Autodesk Fusion 360 part; units mm, degrees
(part 4 of 7)
  spline S86 degree 3 poles (7.7647, -28.9777) (7.9861, -28.9172) (8.1489, -28.7875) (8.2245, -28.6924) (8.2561, -28.6527) (8.2762, -28.616) (8.2885, -28.5883) (8.2955, -28.5727) (8.3002, -28.5603) (8.3276, -28.4858) (8.3447, -28.4393) (8.3614, -28.3763) (8.4396, -28.2255) (8.4953, -28.1181) (8.6034, -27.9308) (8.8139, -27.7502) (8.9794, -27.6083) (9.1711, -27.5171) (9.2695, -27.4797) (9.36, -27.4454) (9.4336, -27.4171) (9.6094, -27.3931) (9.8296, -27.363) (10.1211, -27.3993) (10.2894, -27.4529) (10.6015, -27.5525) (10.6588, -27.6214) (10.7168, -27.6578) (10.8456, -27.7385) (10.8244, -27.7262) (10.8574, -27.741) (10.9657, -27.7894) (11.2076, -27.8277) (11.4806, -27.7163) knots 0.001251 0.001251 0.001251 0.001251 0.25 0.25 0.25 0.35404 0.35404 0.35404 0.412746 0.412746 0.412746 0.449449 0.449449 0.449449 0.475576 0.475576 0.475576 0.496118 0.496118 0.496118 0.514995 0.514995 0.514995 0.538647 0.538647 0.538647 0.582499 0.582499 0.582499 0.679826 0.679826 0.679826 0.99875 0.99875 0.99875 0.99875
  spline S87 degree 3 poles (11.4806, -27.7163) (11.6922, -27.6274) (11.8368, -27.4775) (11.8992, -27.3735) (11.9254, -27.3299) (11.9405, -27.2909) (11.9492, -27.2619) (11.954, -27.2455) (11.9571, -27.2325) (11.9745, -27.1552) (11.9853, -27.1068) (11.9937, -27.0422) (12.0516, -26.8824) (12.0928, -26.7687) (12.1755, -26.5688) (12.3606, -26.3624) (12.5062, -26.2) (12.6843, -26.0846) (12.7771, -26.0347) (12.8623, -25.9889) (12.9316, -25.9512) (13.1027, -25.9045) (13.3171, -25.8459) (13.6108, -25.8438) (13.7847, -25.875) (14.1071, -25.933) (14.173, -25.9939) (14.2352, -26.0223) (14.3734, -26.0856) (14.3508, -26.0762) (14.3854, -26.0865) (14.4991, -26.1203) (14.744, -26.1267) (15.0001, -25.9807) knots 0.001251 0.001251 0.001251 0.001251 0.25 0.25 0.25 0.35404 0.35404 0.35404 0.412746 0.412746 0.412746 0.449449 0.449449 0.449449 0.475576 0.475576 0.475576 0.496118 0.496118 0.496118 0.514995 0.514995 0.514995 0.538647 0.538647 0.538647 0.582499 0.582499 0.582499 0.679826 0.679826 0.679826 0.99875 0.99875 0.99875 0.99875
  spline S88 degree 3 poles (15.0001, -25.9807) (15.1983, -25.8649) (15.322, -25.6975) (15.3704, -25.5861) (15.3906, -25.5395) (15.4006, -25.4989) (15.4053, -25.469) (15.408, -25.4521) (15.4093, -25.4388) (15.4165, -25.3599) (15.421, -25.3105) (15.4208, -25.2453) (15.4573, -25.0794) (15.4834, -24.9613) (15.5393, -24.7523) (15.6959, -24.5234) (15.819, -24.3435) (15.9805, -24.2058) (16.066, -24.1443) (16.1444, -24.0877) (16.2082, -24.0413) (16.3718, -23.9726) (16.5767, -23.8866) (16.8677, -23.8461) (17.0441, -23.8544) (17.3713, -23.8698) (17.4446, -23.9215) (17.51, -23.9416) (17.6553, -23.9863) (17.6316, -23.9799) (17.6673, -23.9856) (17.7844, -24.0044) (18.028, -23.9787) (18.2629, -23.8005) knots 0.001251 0.001251 0.001251 0.001251 0.25 0.25 0.25 0.35404 0.35404 0.35404 0.412746 0.412746 0.412746 0.449449 0.449449 0.449449 0.475576 0.475576 0.475576 0.496118 0.496118 0.496118 0.514995 0.514995 0.514995 0.538647 0.538647 0.538647 0.582499 0.582499 0.582499 0.679826 0.679826 0.679826 0.99875 0.99875 0.99875 0.99875
  spline S89 degree 3 poles (18.2629, -23.8005) (18.4443, -23.6598) (18.5451, -23.4777) (18.5786, -23.361) (18.5925, -23.3122) (18.5971, -23.2705) (18.5979, -23.2403) (18.5984, -23.2232) (18.5979, -23.2099) (18.5947, -23.1307) (18.5927, -23.0811) (18.5841, -23.0165) (18.5986, -22.8472) (18.609, -22.7267) (18.6372, -22.5123) (18.7625, -22.2649) (18.8611, -22.0704) (19.0033, -21.9129) (19.08, -21.8407) (19.1504, -21.7743) (19.2076, -21.72) (19.3608, -21.6306) (19.5527, -21.5185) (19.8359, -21.4404) (20.012, -21.4256) (20.3383, -21.3981) (20.4177, -21.4399) (20.4852, -21.4513) (20.6351, -21.4766) (20.6108, -21.4734) (20.647, -21.4744) (20.7655, -21.4777) (21.0037, -21.4205) (21.2133, -21.2131) knots 0.001251 0.001251 0.001251 0.001251 0.25 0.25 0.25 0.35404 0.35404 0.35404 0.412746 0.412746 0.412746 0.449449 0.449449 0.449449 0.475576 0.475576 0.475576 0.496118 0.496118 0.496118 0.514995 0.514995 0.514995 0.538647 0.538647 0.538647 0.582499 0.582499 0.582499 0.679826 0.679826 0.679826 0.99875 0.99875 0.99875 0.99875
  spline S90 degree 3 poles (21.2133, -21.2131) (21.3747, -21.05) (21.4509, -20.8562) (21.4688, -20.7361) (21.4763, -20.6859) (21.4754, -20.6441) (21.4722, -20.6139) (21.4705, -20.5969) (21.4683, -20.5838) (21.4548, -20.5057) (21.4463, -20.4568) (21.4293, -20.3939) (21.4217, -20.2242) (21.4162, -20.1033) (21.4162, -19.887) (21.5082, -19.6254) (21.5805, -19.4198) (21.701, -19.245) (21.7675, -19.1634) (21.8287, -19.0884) (21.8783, -19.0271) (22.0185, -18.9184) (22.1942, -18.7823) (22.4648, -18.6679) (22.6374, -18.6302) (22.9574, -18.5604) (23.0415, -18.5914) (23.1099, -18.5939) (23.2618, -18.5994) (23.2373, -18.5994) (23.2733, -18.5957) (23.3912, -18.5835) (23.6199, -18.4957) (23.8007, -18.2627) knots 0.001251 0.001251 0.001251 0.001251 0.25 0.25 0.25 0.35404 0.35404 0.35404 0.412746 0.412746 0.412746 0.449449 0.449449 0.449449 0.475576 0.475576 0.475576 0.496118 0.496118 0.496118 0.514995 0.514995 0.514995 0.538647 0.538647 0.538647 0.582499 0.582499 0.582499 0.679826 0.679826 0.679826 0.99875 0.99875 0.99875 0.99875
  spline S91 degree 3 poles (23.8007, -18.2627) (23.9394, -18.0799) (23.9897, -17.8779) (23.9918, -17.7565) (23.9926, -17.7057) (23.9862, -17.6643) (23.9792, -17.6349) (23.9752, -17.6183) (23.9714, -17.6055) (23.9478, -17.5298) (23.933, -17.4825) (23.908, -17.4224) (23.8782, -17.2551) (23.857, -17.136) (23.8287, -16.9215) (23.8858, -16.6502) (23.9307, -16.4368) (24.0273, -16.2478) (24.0826, -16.1582) (24.1335, -16.0759) (24.1747, -16.0086) (24.2995, -15.8826) (24.4559, -15.7247) (24.7092, -15.576) (24.8754, -15.5161) (25.1836, -15.4051) (25.2711, -15.4249) (25.3392, -15.4184) (25.4905, -15.404) (25.4662, -15.4072) (25.5014, -15.3988) (25.6167, -15.3713) (25.832, -15.2544) (25.9808, -14.9999) knots 0.001251 0.001251 0.001251 0.001251 0.25 0.25 0.25 0.35404 0.35404 0.35404 0.412746 0.412746 0.412746 0.449449 0.449449 0.449449 0.475576 0.475576 0.475576 0.496118 0.496118 0.496118 0.514995 0.514995 0.514995 0.538647 0.538647 0.538647 0.582499 0.582499 0.582499 0.679826 0.679826 0.679826 0.99875 0.99875 0.99875 0.99875
  spline S92 degree 3 poles (25.9808, -14.9999) (26.0945, -14.8005) (26.118, -14.5936) (26.1042, -14.473) (26.0984, -14.4226) (26.0867, -14.3824) (26.0759, -14.3541) (26.0698, -14.3382) (26.0643, -14.326) (26.031, -14.2541) (26.0102, -14.2091) (25.9775, -14.1527) (25.9262, -13.9907) (25.8896, -13.8754) (25.8336, -13.6665) (25.8547, -13.39) (25.8714, -13.1726) (25.9425, -12.9726) (25.9857, -12.8766) (26.0253, -12.7883) (26.0574, -12.7162) (26.1647, -12.575) (26.2992, -12.398) (26.5309, -12.2175) (26.6879, -12.1364) (26.9789, -11.9862) (27.0682, -11.9944) (27.135, -11.9791) (27.2831, -11.9451) (27.2594, -11.9514) (27.2932, -11.9385) (27.4039, -11.8962) (27.6021, -11.7522) (27.7164, -11.4804) knots 0.001251 0.001251 0.001251 0.001251 0.25 0.25 0.25 0.35404 0.35404 0.35404 0.412746 0.412746 0.412746 0.449449 0.449449 0.449449 0.475576 0.475576 0.475576 0.496118 0.496118 0.496118 0.514995 0.514995 0.514995 0.538647 0.538647 0.538647 0.582499 0.582499 0.582499 0.679826 0.679826 0.679826 0.99875 0.99875 0.99875 0.99875
  spline S93 degree 3 poles (27.7164, -11.4804) (27.8031, -11.2679) (27.7994, -11.0597) (27.77, -10.9419) (27.7577, -10.8927) (27.7408, -10.8543) (27.7264, -10.8277) (27.7182, -10.8127) (27.7112, -10.8014) (27.6688, -10.7344) (27.6423, -10.6925) (27.6025, -10.6409) (27.5305, -10.487) (27.4792, -10.3774) (27.3964, -10.1776) (27.3813, -9.9007) (27.3694, -9.683) (27.4138, -9.4754) (27.4441, -9.3746) (27.4719, -9.2819) (27.4943, -9.2063) (27.5822, -9.0522) (27.6924, -8.8592) (27.8986, -8.65) (28.0437, -8.5492) (28.3126, -8.3622) (28.4022, -8.3586) (28.4664, -8.3347) (28.6088, -8.2817) (28.5861, -8.2911) (28.618, -8.2739) (28.7223, -8.2175) (28.8999, -8.0488) (28.9778, -7.7644) knots 0.001251 0.001251 0.001251 0.001251 0.25 0.25 0.25 0.35404 0.35404 0.35404 0.412746 0.412746 0.412746 0.449449 0.449449 0.449449 0.475576 0.475576 0.475576 0.496118 0.496118 0.496118 0.514995 0.514995 0.514995 0.538647 0.538647 0.538647 0.582499 0.582499 0.582499 0.679826 0.679826 0.679826 0.99875 0.99875 0.99875 0.99875
  spline S94 degree 3 poles (28.9778, -7.7644) (29.036, -7.5424) (29.0052, -7.3365) (28.9606, -7.2236) (28.942, -7.1764) (28.9203, -7.1406) (28.9025, -7.1161) (28.8924, -7.1022) (28.884, -7.0919) (28.8332, -7.031) (28.8015, -6.993) (28.7553, -6.947) (28.6638, -6.8038) (28.5987, -6.7019) (28.4905, -6.5146) (28.4393, -6.242) (28.3991, -6.0278) (28.4161, -5.8162) (28.4329, -5.7122) (28.4484, -5.6167) (28.4607, -5.5388) (28.5278, -5.3746) (28.6119, -5.1689) (28.789, -4.9345) (28.9196, -4.8156) (29.1619, -4.5951) (29.2503, -4.5799) (29.3108, -4.5478) (29.445, -4.4767) (29.4238, -4.4889) (29.4531, -4.4677) (29.5491, -4.3982) (29.7033, -4.2078) (29.7434, -3.9157) knots 0.001251 0.001251 0.001251 0.001251 0.25 0.25 0.25 0.35404 0.35404 0.35404 0.412746 0.412746 0.412746 0.449449 0.449449 0.449449 0.475576 0.475576 0.475576 0.496118 0.496118 0.496118 0.514995 0.514995 0.514995 0.538647 0.538647 0.538647 0.582499 0.582499 0.582499 0.679826 0.679826 0.679826 0.99875 0.99875 0.99875 0.99875
  spline S95 degree 3 poles (29.7434, -3.9157) (29.7721, -3.6879) (29.7146, -3.4878) (29.6557, -3.3817) (29.6311, -3.3373) (29.6049, -3.3046) (29.584, -3.2827) (29.5723, -3.2703) (29.5626, -3.2612) (29.5043, -3.2074) (29.4679, -3.1738) (29.4161, -3.1342) (29.3067, -3.0042) (29.2288, -2.9117) (29.097, -2.7401) (29.0108, -2.4766) (28.943, -2.2694) (28.9321, -2.0574) (28.9353, -1.9521) (28.9382, -1.8554) (28.9402, -1.7765) (28.9853, -1.605) (29.0418, -1.39) (29.1868, -1.1346) (29.3008, -0.9996) (29.5122, -0.7494) (29.5978, -0.7228) (29.6536, -0.6831) (29.7775, -0.595) (29.758, -0.61) (29.7843, -0.5851) (29.8704, -0.5036) (29.9984, -0.2947) (30, 0.0001) knots 0.001251 0.001251 0.001251 0.001251 0.25 0.25 0.25 0.35404 0.35404 0.35404 0.412746 0.412746 0.412746 0.449449 0.449449 0.449449 0.475576 0.475576 0.475576 0.496118 0.496118 0.496118 0.514995 0.514995 0.514995 0.538647 0.538647 0.538647 0.582499 0.582499 0.582499 0.679826 0.679826 0.679826 0.99875 0.99875 0.99875 0.99875
  point P0 (31.1223, 4.5793)
  point P1 (30.9354, 4.999)
  point P2 (30.6966, 5.3433)
  point P3 (30.4412, 5.5983)
  point P4 (30.2076, 5.7661)
  point P5 (30.0296, 5.8646)
  point P6 (29.9305, 5.9238)
  point P7 (29.914, 5.9503)
  point P8 (29.9191, 5.981)
  point P9 (29.988, 6.0737)
  point P10 (30.1148, 6.2328)
  point P11 (30.2664, 6.4772)
  point P12 (30.4047, 6.8105)
  point P13 (30.4937, 7.22)
  point P14 (30.5057, 7.6793)
  point P15 (30.2584, 8.6024)
  point P16 (30.0182, 8.9941)
  point P17 (29.7365, 9.3043)
  point P18 (29.4501, 9.5238)
  point P19 (29.1966, 9.6597)
  point P20 (29.0072, 9.734)
  point P21 (28.9012, 9.7798)
  point P22 (28.8814, 9.8039)
  point P23 (28.8825, 9.8351)
  point P24 (28.9387, 9.9359)
  point P25 (29.0436, 10.1102)
  point P26 (29.162, 10.3724)
  point P27 (29.2557, 10.7208)
  point P28 (29.2904, 11.1384)
  point P29 (29.2424, 11.5954)
  point P30 (28.8766, 12.4783)
  point P31 (28.5875, 12.8354)
  point P32 (28.2676, 13.1061)
  point P33 (27.955, 13.2863)
  point P34 (27.686, 13.388)
  point P35 (27.4885, 13.437)
  point P36 (27.3775, 13.4685)
  point P37 (27.3546, 13.4898)
  point P38 (27.3517, 13.5209)
  point P39 (27.3942, 13.6282)
  point P40 (27.4755, 13.8147)
  point P41 (27.5587, 14.09)
  point P42 (27.606, 14.4477)
  point P43 (27.586, 14.8663)
  point P44 (27.4787, 15.3131)
  point P45 (27.0009, 16.1407)
  point P46 (26.6675, 16.457)
  point P47 (26.3151, 16.6836)
  point P48 (25.9817, 16.8215)
  point P49 (25.7016, 16.8872)
  point P50 (25.4995, 16.91)
  point P51 (25.3853, 16.9268)
  point P52 (25.3598, 16.9449)
  point P53 (25.3528, 16.9753)
  point P54 (25.381, 17.0873)
  point P55 (25.4373, 17.2828)
  point P56 (25.4838, 17.5666)
  point P57 (25.484, 17.9275)
  point P58 (25.4095, 18.3398)
  point P59 (25.2449, 18.7687)
  point P60 (24.6631, 19.527)
  point P61 (24.2913, 19.797)
  point P62 (23.9123, 19.9757)
  point P63 (23.5637, 20.0689)
  point P64 (23.2775, 20.0974)
  point P65 (23.0741, 20.0937)
  point P66 (22.9587, 20.0954)
  point P67 (22.9311, 20.11)
  point P68 (22.9202, 20.1393)
  point P69 (22.9335, 20.254)
  point P70 (22.9638, 20.4551)
  point P71 (22.9729, 20.7426)
  point P72 (22.926, 21.1004)
  point P73 (22.7983, 21.4995)
  point P74 (22.5791, 21.9033)
  point P75 (21.9033, 22.5791)
  point P76 (21.4995, 22.7983)
  point P77 (21.1004, 22.926)
  point P78 (20.7426, 22.9729)
  point P79 (20.4551, 22.9638)
  point P80 (20.254, 22.9335)
  point P81 (20.1393, 22.9202)
  point P82 (20.11, 22.9311)
  point P83 (20.0954, 22.9587)
  point P84 (20.0937, 23.0741)
  point P85 (20.0974, 23.2775)
  point P86 (20.0689, 23.5637)
  point P87 (19.9757, 23.9123)
  point P88 (19.797, 24.2914)
  point P89 (19.527, 24.6631)
  point P90 (18.7687, 25.2449)
  point P91 (18.3398, 25.4095)
  point P92 (17.9275, 25.484)
  point P93 (17.5666, 25.4838)
  point P94 (17.2828, 25.4373)
  point P95 (17.0873, 25.381)
  point P96 (16.9753, 25.3528)
  point P97 (16.9449, 25.3598)
  point P98 (16.9268, 25.3853)
  point P99 (16.91, 25.4995)
  point P100 (16.8872, 25.7016)
  point P101 (16.8215, 25.9817)
  point P102 (16.6836, 26.3151)
  point P103 (16.457, 26.6676)
  point P104 (16.1407, 27.0009)
  point P105 (15.3131, 27.4787)
  point P106 (14.8663, 27.5859)
  point P107 (14.4477, 27.606)
  point P108 (14.09, 27.5587)
  point P109 (13.8147, 27.4755)
  point P110 (13.6282, 27.3942)
  point P111 (13.5209, 27.3517)
  point P112 (13.4898, 27.3546)
  point P113 (13.4685, 27.3775)
  point P114 (13.437, 27.4885)
  point P115 (13.388, 27.686)
  point P116 (13.2863, 27.955)
  point P117 (13.1061, 28.2676)
  point P118 (12.8354, 28.5875)
  point P119 (12.4783, 28.8766)
  point P120 (11.5954, 29.2424)
  point P121 (11.1384, 29.2904)
  point P122 (10.7208, 29.2557)
  point P123 (10.3724, 29.162)
  point P124 (10.1102, 29.0436)
  point P125 (9.9359, 28.9387)
  point P126 (9.8351, 28.8825)
  point P127 (9.8039, 28.8814)
  point P128 (9.7798, 28.9012)
  point P129 (9.734, 29.0072)
  point P130 (9.6597, 29.1966)
  point P131 (9.5238, 29.4501)
  point P132 (9.3043, 29.7365)
  point P133 (8.9942, 30.0183)
  point P134 (8.6024, 30.2584)
  point P135 (7.6793, 30.5057)
  point P136 (7.22, 30.4936)
  point P137 (6.8105, 30.4047)
  point P138 (6.4772, 30.2664)
  point P139 (6.2328, 30.1148)
  point P140 (6.0737, 29.988)
  point P141 (5.981, 29.9191)
  point P142 (5.9503, 29.914)
  point P143 (5.9238, 29.9305)
  point P144 (5.8646, 30.0296)
  point P145 (5.7661, 30.2076)
  point P146 (5.5983, 30.4412)
  point P147 (5.3433, 30.6966)
  point P148 (4.999, 30.9355)
  point P149 (4.5793, 31.1223)
  point P150 (3.6318, 31.2471)
  point P151 (3.178, 31.1751)
  point P152 (2.7836, 31.0335)
  point P153 (2.4712, 30.8529)
  point P154 (2.2487, 30.6707)
  point P155 (2.1075, 30.5242)
  point P156 (2.0246, 30.4439)
  point P157 (1.9948, 30.4347)
  point P158 (1.9664, 30.4477)
  point P159 (1.8947, 30.5382)
  point P160 (1.7739, 30.7018)
  point P161 (1.577, 30.9115)
  point P162 (1.2909, 31.1314)
  point P163 (0.9184, 31.3233)
  point P164 (0.4779, 31.4538)
  point P165 (-0.4779, 31.4538)
  point P166 (-0.9184, 31.3233)
  point P167 (-1.2909, 31.1314)
  point P168 (-1.577, 30.9115)
  point P169 (-1.7739, 30.7018)
  point P170 (-1.8947, 30.5382)
  point P171 (-1.9664, 30.4477)
  point P172 (-1.9948, 30.4347)
  point P173 (-2.0246, 30.4439)
  point P174 (-2.1075, 30.5242)
  point P175 (-2.2487, 30.6707)
  point P176 (-2.4712, 30.8529)
  point P177 (-2.7836, 31.0335)
  point P178 (-3.178, 31.1752)
  point P179 (-3.6318, 31.2471)
  point P180 (-4.5793, 31.1223)
  point P181 (-4.999, 30.9354)
  point P182 (-5.3433, 30.6966)
  point P183 (-5.5983, 30.4412)
  point P184 (-5.7661, 30.2076)
  point P185 (-5.8646, 30.0296)
  point P186 (-5.9238, 29.9305)
  point P187 (-5.9503, 29.914)
  point P188 (-5.981, 29.9191)
  point P189 (-6.0737, 29.988)
  point P190 (-6.2328, 30.1148)
  point P191 (-6.4772, 30.2664)
  point P192 (-6.8105, 30.4047)
  point P193 (-7.22, 30.4937)
  point P194 (-7.6793, 30.5057)
  point P195 (-8.6024, 30.2584)
  point P196 (-8.9941, 30.0182)
  point P197 (-9.3043, 29.7365)
  point P198 (-9.5238, 29.4501)
  point P199 (-9.6597, 29.1966)
  point P200 (-9.734, 29.0072)
  point P201 (-9.7798, 28.9012)
  point P202 (-9.8039, 28.8814)
  point P203 (-9.8351, 28.8825)
  point P204 (-9.9359, 28.9387)
  point P205 (-10.1102, 29.0436)
  point P206 (-10.3724, 29.162)
  point P207 (-10.7208, 29.2557)
  point P208 (-11.1384, 29.2904)
  point P209 (-11.5954, 29.2424)
  point P210 (-12.4783, 28.8766)
  point P211 (-12.8354, 28.5875)
  point P212 (-13.1061, 28.2676)
  point P213 (-13.2863, 27.955)
  point P214 (-13.388, 27.686)
  point P215 (-13.437, 27.4885)
  point P216 (-13.4685, 27.3775)
  point P217 (-13.4898, 27.3546)
  point P218 (-13.5209, 27.3517)
  point P219 (-13.6282, 27.3942)
  point P220 (-13.8147, 27.4755)
  point P221 (-14.09, 27.5587)
  point P222 (-14.4477, 27.606)
  point P223 (-14.8663, 27.586)
  point P224 (-15.3131, 27.4787)
  point P225 (-16.1407, 27.0009)
  point P226 (-16.457, 26.6675)
  point P227 (-16.6836, 26.3151)
  point P228 (-16.8215, 25.9817)
  point P229 (-16.8872, 25.7016)
  point P230 (-16.91, 25.4995)
  point P231 (-16.9268, 25.3853)
  point P232 (-16.9449, 25.3598)
  point P233 (-16.9753, 25.3528)
  point P234 (-17.0873, 25.381)
  point P235 (-17.2828, 25.4373)
  point P236 (-17.5666, 25.4838)
  point P237 (-17.9275, 25.484)
  point P238 (-18.3398, 25.4095)
  point P239 (-18.7687, 25.2449)
  point P240 (-19.527, 24.6631)
  point P241 (-19.797, 24.2913)
  point P242 (-19.9757, 23.9123)
  point P243 (-20.0689, 23.5637)
  point P244 (-20.0974, 23.2775)
  point P245 (-20.0937, 23.0741)
  point P246 (-20.0954, 22.9587)
  point P247 (-20.11, 22.9311)
  point P248 (-20.1393, 22.9202)
  point P249 (-20.254, 22.9335)
  point P250 (-20.4551, 22.9638)
  point P251 (-20.7426, 22.9729)
  point P252 (-21.1004, 22.926)
  point P253 (-21.4995, 22.7983)
  point P254 (-21.9033, 22.5791)
  point P255 (-22.5791, 21.9033)
  point P256 (-22.7983, 21.4995)
  point P257 (-22.926, 21.1004)
  point P258 (-22.9729, 20.7426)
  point P259 (-22.9638, 20.4551)
  point P260 (-22.9335, 20.254)
  point P261 (-22.9202, 20.1393)
  point P262 (-22.9311, 20.11)
  point P263 (-22.9587, 20.0954)
  point P264 (-23.0741, 20.0937)
  point P265 (-23.2775, 20.0974)
  point P266 (-23.5637, 20.0689)
  point P267 (-23.9123, 19.9757)
  point P268 (-24.2914, 19.797)
  point P269 (-24.6631, 19.527)
  point P270 (-25.2449, 18.7687)
  point P271 (-25.4095, 18.3398)
  point P272 (-25.484, 17.9275)
  point P273 (-25.4838, 17.5666)
  point P274 (-25.4373, 17.2828)
  point P275 (-25.381, 17.0873)
  point P276 (-25.3528, 16.9753)
  point P277 (-25.3598, 16.9449)
  point P278 (-25.3853, 16.9268)
  point P279 (-25.4995, 16.91)
  point P280 (-25.7016, 16.8872)
  point P281 (-25.9817, 16.8215)
  point P282 (-26.3151, 16.6836)
  point P283 (-26.6676, 16.457)
  point P284 (-27.0009, 16.1407)
  point P285 (-27.4787, 15.3131)
  point P286 (-27.5859, 14.8663)
  point P287 (-27.606, 14.4477)
  point P288 (-27.5587, 14.09)
  point P289 (-27.4755, 13.8147)
  point P290 (-27.3942, 13.6282)
  point P291 (-27.3517, 13.5209)
  point P292 (-27.3546, 13.4898)
  point P293 (-27.3775, 13.4685)
  point P294 (-27.4885, 13.437)
  point P295 (-27.686, 13.388)
  point P296 (-27.955, 13.2863)
  point P297 (-28.2676, 13.1061)
  point P298 (-28.5875, 12.8354)
  point P299 (-28.8766, 12.4783)
  point P300 (-29.2424, 11.5954)
  point P301 (-29.2904, 11.1384)
  point P302 (-29.2557, 10.7208)
  point P303 (-29.162, 10.3724)
  point P304 (-29.0436, 10.1102)
  point P305 (-28.9387, 9.9359)
  point P306 (-28.8825, 9.8351)
  point P307 (-28.8814, 9.8039)
  point P308 (-28.9012, 9.7798)
  point P309 (-29.0072, 9.734)
  point P310 (-29.1966, 9.6597)
  point P311 (-29.4501, 9.5238)
  point P312 (-29.7365, 9.3043)
  point P313 (-30.0183, 8.9942)
  point P314 (-30.2584, 8.6024)
  point P315 (-30.5057, 7.6793)
  point P316 (-30.4936, 7.22)
  point P317 (-30.4047, 6.8105)
  point P318 (-30.2664, 6.4772)
  point P319 (-30.1148, 6.2328)
  point P320 (-29.988, 6.0737)
  point P321 (-29.9191, 5.981)
  point P322 (-29.914, 5.9503)
  point P323 (-29.9305, 5.9238)
  point P324 (-30.0296, 5.8646)
  point P325 (-30.2076, 5.7661)
  point P326 (-30.4412, 5.5983)
  point P327 (-30.6966, 5.3433)
  point P328 (-30.9355, 4.999)
  point P329 (-31.1223, 4.5793)
  point P330 (-31.2471, 3.6318)
  point P331 (-31.1751, 3.178)
  point P332 (-31.0335, 2.7836)
  point P333 (-30.8529, 2.4712)
  point P334 (-30.6707, 2.2487)
  point P335 (-30.5242, 2.1075)
  point P336 (-30.4439, 2.0246)
  point P337 (-30.4347, 1.9948)
  point P338 (-30.4477, 1.9664)
  point P339 (-30.5382, 1.8947)
  point P340 (-30.7018, 1.7739)
  point P341 (-30.9115, 1.577)
  point P342 (-31.1314, 1.2909)
  point P343 (-31.3233, 0.9184)
  point P344 (-31.4538, 0.4779)
  point P345 (-31.4538, -0.4779)
  point P346 (-31.3233, -0.9184)
  point P347 (-31.1314, -1.2909)
  point P348 (-30.9115, -1.577)
  point P349 (-30.7018, -1.7739)
  point P350 (-30.5382, -1.8947)
  point P351 (-30.4477, -1.9664)
  point P352 (-30.4347, -1.9948)
  point P353 (-30.4439, -2.0246)
  point P354 (-30.5242, -2.1075)
  point P355 (-30.6707, -2.2487)
  point P356 (-30.8529, -2.4712)
  point P357 (-31.0335, -2.7836)
  point P358 (-31.1752, -3.178)
  point P359 (-31.2471, -3.6318)
  point P360 (-31.1223, -4.5793)
  point P361 (-30.9354, -4.999)
  point P362 (-30.6966, -5.3433)
  point P363 (-30.4412, -5.5983)
  point P364 (-30.2076, -5.7661)
  point P365 (-30.0296, -5.8646)
  point P366 (-29.9305, -5.9238)
  point P367 (-29.914, -5.9503)
  point P368 (-29.9191, -5.981)
  point P369 (-29.988, -6.0737)
  point P370 (-30.1148, -6.2328)
  point P371 (-30.2664, -6.4772)
  point P372 (-30.4047, -6.8105)
  point P373 (-30.4937, -7.22)
  point P374 (-30.5057, -7.6793)
  point P375 (-30.2584, -8.6024)
  point P376 (-30.0182, -8.9941)
  point P377 (-29.7365, -9.3043)
  point P378 (-29.4501, -9.5238)
  point P379 (-29.1966, -9.6597)
  point P380 (-29.0072, -9.734)
  point P381 (-28.9012, -9.7798)
  point P382 (-28.8814, -9.8039)
  point P383 (-28.8825, -9.8351)
  point P384 (-28.9387, -9.9359)
  point P385 (-29.0436, -10.1102)
  point P386 (-29.162, -10.3724)
  point P387 (-29.2557, -10.7208)
  point P388 (-29.2904, -11.1384)
  point P389 (-29.2424, -11.5954)
  point P390 (-28.8766, -12.4783)
  point P391 (-28.5875, -12.8354)
  point P392 (-28.2676, -13.1061)
  point P393 (-27.955, -13.2863)
  point P394 (-27.686, -13.388)
  point P395 (-27.4885, -13.437)
  point P396 (-27.3775, -13.4685)
  point P397 (-27.3546, -13.4898)
  point P398 (-27.3517, -13.5209)
  point P399 (-27.3942, -13.6282)
  point P400 (-27.4755, -13.8147)
  point P401 (-27.5587, -14.09)
  point P402 (-27.606, -14.4477)
  point P403 (-27.586, -14.8663)
  point P404 (-27.4787, -15.3131)
  point P405 (-27.0009, -16.1407)
  point P406 (-26.6675, -16.457)
  point P407 (-26.3151, -16.6836)
  point P408 (-25.9817, -16.8215)
  point P409 (-25.7016, -16.8872)
  point P410 (-25.4995, -16.91)
  point P411 (-25.3853, -16.9268)
  point P412 (-25.3598, -16.9449)
  point P413 (-25.3528, -16.9753)
  point P414 (-25.381, -17.0873)
  point P415 (-25.4373, -17.2828)
  point P416 (-25.4838, -17.5666)
  point P417 (-25.484, -17.9275)
  point P418 (-25.4095, -18.3398)
  point P419 (-25.2449, -18.7687)
  point P420 (-24.6631, -19.527)
  point P421 (-24.2913, -19.797)
  point P422 (-23.9123, -19.9757)
  point P423 (-23.5637, -20.0689)
  point P424 (-23.2775, -20.0974)
  point P425 (-23.0741, -20.0937)
  point P426 (-22.9587, -20.0954)
  point P427 (-22.9311, -20.11)
  point P428 (-22.9202, -20.1393)
  point P429 (-22.9335, -20.254)
  point P430 (-22.9638, -20.4551)
  point P431 (-22.9729, -20.7426)
  point P432 (-22.926, -21.1004)
  point P433 (-22.7983, -21.4995)
  point P434 (-22.5791, -21.9033)
  point P435 (-21.9033, -22.5791)
  point P436 (-21.4995, -22.7983)
  point P437 (-21.1004, -22.926)
  point P438 (-20.7426, -22.9729)
  point P439 (-20.4551, -22.9638)
  point P440 (-20.254, -22.9335)
  point P441 (-20.1393, -22.9202)
  point P442 (-20.11, -22.9311)
  point P443 (-20.0954, -22.9587)
  point P444 (-20.0937, -23.0741)
  point P445 (-20.0974, -23.2775)
  point P446 (-20.0689, -23.5637)
  point P447 (-19.9757, -23.9123)
  point P448 (-19.797, -24.2914)
  point P449 (-19.527, -24.6631)
  point P450 (-18.7687, -25.2449)
  point P451 (-18.3398, -25.4095)
  point P452 (-17.9275, -25.484)
  point P453 (-17.5666, -25.4838)
  point P454 (-17.2828, -25.4373)
  point P455 (-17.0873, -25.381)
  point P456 (-16.9753, -25.3528)
  point P457 (-16.9449, -25.3598)
  point P458 (-16.9268, -25.3853)
  point P459 (-16.91, -25.4995)
  point P460 (-16.8872, -25.7016)
  point P461 (-16.8215, -25.9817)
  point P462 (-16.6836, -26.3151)
  point P463 (-16.457, -26.6676)
  point P464 (-16.1407, -27.0009)
  point P465 (-15.3131, -27.4787)
  point P466 (-14.8663, -27.5859)
  point P467 (-14.4477, -27.606)
  point P468 (-14.09, -27.5587)
  point P469 (-13.8147, -27.4755)
  point P470 (-13.6282, -27.3942)
  point P471 (-13.5209, -27.3517)
  point P472 (-13.4898, -27.3546)
  point P473 (-13.4685, -27.3775)
  point P474 (-13.437, -27.4885)
  point P475 (-13.388, -27.686)
  point P476 (-13.2863, -27.955)
  point P477 (-13.1061, -28.2676)
  point P478 (-12.8354, -28.5875)
  point P479 (-12.4783, -28.8766)
  point P480 (-11.5954, -29.2424)
  point P481 (-11.1384, -29.2904)
  point P482 (-10.7208, -29.2557)
  point P483 (-10.3724, -29.162)
  point P484 (-10.1102, -29.0436)
  point P485 (-9.9359, -28.9387)
  point P486 (-9.8351, -28.8825)
  point P487 (-9.8039, -28.8814)
  point P488 (-9.7798, -28.9012)
  point P489 (-9.734, -29.0072)
  point P490 (-9.6597, -29.1966)
  point P491 (-9.5238, -29.4501)
  point P492 (-9.3043, -29.7365)
  point P493 (-8.9942, -30.0183)
  point P494 (-8.6024, -30.2584)
  point P495 (-7.6793, -30.5057)
  point P496 (-7.22, -30.4936)
  point P497 (-6.8105, -30.4047)
  point P498 (-6.4772, -30.2664)
  point P499 (-6.2328, -30.1148)
  point P500 (-6.0737, -29.988)
  point P501 (-5.981, -29.9191)
  point P502 (-5.9503, -29.914)
  point P503 (-5.9238, -29.9305)
  point P504 (-5.8646, -30.0296)
  point P505 (-5.7661, -30.2076)
  point P506 (-5.5983, -30.4412)
  point P507 (-5.3433, -30.6966)
  point P508 (-4.999, -30.9355)
  point P509 (-4.5793, -31.1223)
  point P510 (-3.6318, -31.2471)
  point P511 (-3.178, -31.1751)
  point P512 (-2.7836, -31.0335)
  point P513 (-2.4712, -30.8529)
  point P514 (-2.2487, -30.6707)
  point P515 (-2.1075, -30.5242)
  point P516 (-2.0246, -30.4439)
  point P517 (-1.9948, -30.4347)
  point P518 (-1.9664, -30.4477)
  point P519 (-1.8947, -30.5382)
  point P520 (-1.7739, -30.7018)
  point P521 (-1.577, -30.9115)
  point P522 (-1.2909, -31.1314)
  point P523 (-0.9184, -31.3233)
  point P524 (-0.4779, -31.4538)
  point P525 (0.4779, -31.4538)
  point P526 (0.9184, -31.3233)
  point P527 (1.2909, -31.1314)
  point P528 (1.577, -30.9115)
  point P529 (1.7739, -30.7018)
  point P530 (1.8947, -30.5382)
  point P531 (1.9664, -30.4477)
  point P532 (1.9948, -30.4347)
  point P533 (2.0246, -30.4439)
  point P534 (2.1075, -30.5242)
  point P535 (2.2487, -30.6707)
  point P536 (2.4712, -30.8529)
  point P537 (2.7836, -31.0335)
  point P538 (3.178, -31.1752)
  point P539 (3.6318, -31.2471)
  point P540 (4.5793, -31.1223)
  point P541 (4.999, -30.9354)
  point P542 (5.3433, -30.6966)
  point P543 (5.5983, -30.4412)
  point P544 (5.7661, -30.2076)
  point P545 (5.8646, -30.0296)
  point P546 (5.9238, -29.9305)
  point P547 (5.9503, -29.914)
  point P548 (5.981, -29.9191)
  point P549 (6.0737, -29.988)
  point P550 (6.2328, -30.1148)
  point P551 (6.4772, -30.2664)
  point P552 (6.8105, -30.4047)
  point P553 (7.22, -30.4937)
  point P554 (7.6793, -30.5057)
  point P555 (8.6024, -30.2584)
  point P556 (8.9941, -30.0182)
  point P557 (9.3043, -29.7365)
  point P558 (9.5238, -29.4501)
  point P559 (9.6597, -29.1966)
  point P560 (9.734, -29.0072)
  point P561 (9.7798, -28.9012)
  point P562 (9.8039, -28.8814)
  point P563 (9.8351, -28.8825)
  point P564 (9.9359, -28.9387)
  point P565 (10.1102, -29.0436)
  point P566 (10.3724, -29.162)
  point P567 (10.7208, -29.2557)
  point P568 (11.1384, -29.2904)
  point P569 (11.5954, -29.2424)
  point P570 (12.4783, -28.8766)
  point P571 (12.8354, -28.5875)
  point P572 (13.1061, -28.2676)
  point P573 (13.2863, -27.955)
  point P574 (13.388, -27.686)
  point P575 (13.437, -27.4885)
  point P576 (13.4685, -27.3775)
  point P577 (13.4898, -27.3546)
  point P578 (13.5209, -27.3517)
  point P579 (13.6282, -27.3942)
  point P580 (13.8147, -27.4755)
  point P581 (14.09, -27.5587)
  point P582 (14.4477, -27.606)
  point P583 (14.8663, -27.586)
  point P584 (15.3131, -27.4787)
  point P585 (16.1407, -27.0009)
  point P586 (16.457, -26.6675)
  point P587 (16.6836, -26.3151)
  point P588 (16.8215, -25.9817)
  point P589 (16.8872, -25.7016)
  point P590 (16.91, -25.4995)
  point P591 (16.9268, -25.3853)
  point P592 (16.9449, -25.3598)
  point P593 (16.9753, -25.3528)
  point P594 (17.0873, -25.381)
  point P595 (17.2828, -25.4373)
  point P596 (17.5666, -25.4838)
  point P597 (17.9275, -25.484)
  point P598 (18.3398, -25.4095)
  point P599 (18.7687, -25.2449)
  point P600 (19.527, -24.6631)
  point P601 (19.797, -24.2913)
  point P602 (19.9757, -23.9123)
  point P603 (20.0689, -23.5637)
  point P604 (20.0974, -23.2775)
  point P605 (20.0937, -23.0741)
  point P606 (20.0954, -22.9587)
  point P607 (20.11, -22.9311)
  point P608 (20.1393, -22.9202)
  point P609 (20.254, -22.9335)
  point P610 (20.4551, -22.9638)
  point P611 (20.7426, -22.9729)
  point P612 (21.1004, -22.926)
  point P613 (21.4995, -22.7983)
  point P614 (21.9033, -22.5791)
  point P615 (22.5791, -21.9033)
  point P616 (22.7983, -21.4995)
  point P617 (22.926, -21.1004)
  point P618 (22.9729, -20.7426)
  point P619 (22.9638, -20.4551)
  point P620 (22.9335, -20.254)
  point P621 (22.9202, -20.1393)
  point P622 (22.9311, -20.11)
  point P623 (22.9587, -20.0954)
  point P624 (23.0741, -20.0937)
  point P625 (23.2775, -20.0974)
  point P626 (23.5637, -20.0689)
  point P627 (23.9123, -19.9757)
  point P628 (24.2914, -19.797)
  point P629 (24.6631, -19.527)
  point P630 (25.2449, -18.7687)
  point P631 (25.4095, -18.3398)
  point P632 (25.484, -17.9275)
  point P633 (25.4838, -17.5666)
  point P634 (25.4373, -17.2828)
  point P635 (25.381, -17.0873)
  point P636 (25.3528, -16.9753)
  point P637 (25.3598, -16.9449)
  point P638 (25.3853, -16.9268)
  point P639 (25.4995, -16.91)
  point P640 (25.7016, -16.8872)
  point P641 (25.9817, -16.8215)
  point P642 (26.3151, -16.6836)
  point P643 (26.6676, -16.457)
  point P644 (27.0009, -16.1407)
  point P645 (27.4787, -15.3131)
  point P646 (27.5859, -14.8663)
  point P647 (27.606, -14.4477)
  point P648 (27.5587, -14.09)
  point P649 (27.4755, -13.8147)
  point P650 (27.3942, -13.6282)
  point P651 (27.3517, -13.5209)
  point P652 (27.3546, -13.4898)
  point P653 (27.3775, -13.4685)
  point P654 (27.4885, -13.437)
  point P655 (27.686, -13.388)
  point P656 (27.955, -13.2863)
  point P657 (28.2676, -13.1061)
  point P658 (28.5875, -12.8354)
  point P659 (28.8766, -12.4783)
  point P660 (29.2424, -11.5954)
  point P661 (29.2904, -11.1384)
  point P662 (29.2557, -10.7208)
  point P663 (29.162, -10.3724)
  point P664 (29.0436, -10.1102)
  point P665 (28.9387, -9.9359)
  point P666 (28.8825, -9.8351)
  point P667 (28.8814, -9.8039)
  point P668 (28.9012, -9.7798)
  point P669 (29.0072, -9.734)
  point P670 (29.1966, -9.6597)
  point P671 (29.4501, -9.5238)
  point P672 (29.7365, -9.3043)
  point P673 (30.0183, -8.9942)
  point P674 (30.2584, -8.6024)
  point P675 (30.5057, -7.6793)
  point P676 (30.4936, -7.22)
  point P677 (30.4047, -6.8105)
  point P678 (30.2664, -6.4772)
  point P679 (30.1148, -6.2328)
  point P680 (29.988, -6.0737)
  point P681 (29.9191, -5.981)
  point P682 (29.914, -5.9503)
  point P683 (29.9305, -5.9238)
  point P684 (30.0296, -5.8646)
  point P685 (30.2076, -5.7661)
  point P686 (30.4412, -5.5983)
  point P687 (30.6966, -5.3433)
  point P688 (30.9355, -4.999)
  point P689 (31.1223, -4.5793)
  point P690 (31.2471, -3.6318)
  point P691 (31.1751, -3.178)
  point P692 (31.0335, -2.7836)
  point P693 (30.8529, -2.4712)
  point P694 (30.6707, -2.2487)
  point P695 (30.5242, -2.1075)
  point P696 (30.4439, -2.0246)
  point P697 (30.4347, -1.9948)
  point P698 (30.4477, -1.9664)
  point P699 (30.5382, -1.8947)
  point P700 (30.7018, -1.7739)
  point P701 (30.9115, -1.577)
  point P702 (31.1314, -1.2909)
  point P703 (31.3233, -0.9184)
  point P704 (31.4538, -0.4779)
  dimension "d1" = 60.734
  dimension "d2" = 1.266
  dimension "d3" = 7.5
  dimension "d4" = 0.5
  dimension "d5" = 1
  dimension "d6" = 1.5
  dimension "d7" = 2
  dimension "d8" = 2.5
  dimension "d9" = 3
  dimension "d10" = 3.5
  dimension "d12" = 4
  dimension "d13" = 4.5
  dimension "d14" = 5
  dimension "d15" = 5.5
  dimension "d16" = 6
  dimension "d17" = 6.5
  dimension "d18" = 7
  dimension "d21" = 0.5
  dimension "d22" = 24.5
  dimension "d25" = 0.5
  dimension "d26" = 49
  dimension "d27" = 73.5
  dimension "d28" = 0.5
  dimension "d29" = 98
  dimension "d30" = 0.5
  dimension "d31" = 0.5
  dimension "d32" = 122.5
  dimension "d33" = 147
  dimension "d34" = 0.5
  dimension "d35" = 171.5
  dimension "d36" = 0.5
  dimension "d37" = 0.5
  dimension "d38" = 164
  dimension "d39" = 3.75
  dimension "d40" = 3.75
  dimension "d41" = 0.5
  dimension "d42" = 40.5
  dimension "d43" = 0.5
  dimension "d44" = 65
  dimension "d45" = 0.5
  dimension "d46" = 89.5
  dimension "d47" = 0.5
  dimension "d48" = 114
  dimension "d49" = 0.5
  dimension "d50" = 138.5
  dimension "d51" = 0.5
  dimension "d52" = 163
  dimension "d53" = 0.5
  dimension "d56" = 367.5
  dimension "d57" = 0.5
  dimension "d58" = 0.5
  dimension "d60" = 360
  dimension "d61" = -1.5
  constraint coincident A0.centre L0.start
  constraint tangent A0 A1
  constraint horizontal A0.centre A1.centre
  constraint horizontal L1
  constraint coincident A1.centre A2
  constraint horizontal L3
  constraint horizontal L5
  constraint horizontal L7
  constraint horizontal L9
  constraint horizontal L11
  constraint horizontal L13
  constraint horizontal L15
  constraint horizontal L17
  constraint horizontal L19
  constraint horizontal L21
  constraint horizontal L23
  constraint horizontal L25
  constraint horizontal L27
  constraint horizontal L29
  constraint coincident A2 L28.end
  constraint coincident A2 L26.end
  constraint coincident A2 L24.end
  constraint coincident A2 L22.end
  constraint coincident A2 L20.end
  constraint coincident A2 L18.end
  constraint coincident A2 L16.end
  constraint coincident A2 L14.end
  constraint coincident A2 L12.end
  constraint coincident A2 L10.end
  constraint coincident A2 L8.end
  constraint coincident A2 L6.end
  constraint horizontal L30
  constraint coincident A2 L2.end
  constraint horizontal L32
  constraint horizontal L33
  constraint horizontal L35
  constraint horizontal L37
  constraint horizontal L39
  constraint horizontal L41
  constraint horizontal L43
  constraint horizontal L45
  constraint horizontal L47
  constraint horizontal L49
  constraint coincident A2 L48.end
  constraint horizontal L51
  constraint horizontal L53
  constraint horizontal L55
  constraint horizontal L57
  constraint horizontal L59
  constraint horizontal L61
  constraint horizontal L63
  constraint horizontal L65
  constraint coincident A2 L64.start
  constraint coincident L0 L64.start
  constraint coincident A1.centre L66.start
  constraint parallel L13 L66
  measures "d1" diameter of A0
  measures "d2" diameter of A1
  measures "d3" angle of L0 L1
  measures "d4" angle of L2 L3
  measures "d5" angle of L4 L5
  measures "d6" angle of L6 L7
  measures "d7" angle of L8 L9
  measures "d8" angle of L10 L11
  measures "d9" angle of L12 L13
  measures "d10" angle of L14 L15
  measures "d12" angle of L16 L17
  measures "d13" angle of L18 L19
  measures "d14" angle of L20 L21
  measures "d15" angle of L22 L23
  measures "d16" angle of L24 L25
  measures "d17" angle of L26 L27
  measures "d18" angle of L28 L29
  measures "d21" distance of L2.end L31.end
  measures "d22" angle of L31 L32
  measures "d25" distance of L4.end L34.end
  measures "d26" angle of L34 L35
  measures "d27" angle of L36 L37
  measures "d28" distance of L6.end L36.end
  measures "d29" angle of L38 L39
  measures "d30" distance of L8.end L38.end
  measures "d31" distance of L10.end L40.end
  measures "d32" angle of L40 L41
  measures "d33" angle of L42 L43
  measures "d34" distance of L12.end L42.end
  measures "d35" angle of L44 L45
  measures "d36" distance of L14.end L44.end
  measures "d37" distance of L16.end L46.end
  measures "d38" angle of L46 L47
  measures "d39" angle of L48 L49
  measures "d40" angle of L50 L51
  measures "d41" distance of L48.end L50.end
  measures "d42" angle of L52 L53
  measures "d43" distance of L18.end L52.end
  measures "d44" angle of L54 L55
  measures "d45" distance of L20.end L54.end
  measures "d46" angle of L56 L57
  measures "d47" distance of L22.end L56.end
  measures "d48" angle of L58 L59
  measures "d49" distance of L24.end L58.end
  measures "d50" angle of L60 L61
  measures "d51" distance of L26.end L60.end
  measures "d52" angle of L62 L63
  measures "d53" distance of L28.end L62.end
  measures "d57" distance of L64.start L64.end
  measures "d58" distance of A1.centre L66.end
extrude "Extrude1" add sketch "Sketch1" along normal blind 2.4 contours L0 L2 S48 S49 S50 S51 S52 S53 S54 S55 S56 S57 S58 S59 S60 S61 S62 S63 S64 S65 S66 S67 S68 S69 S70 S71 S72 S73 S74 S75 S76 S77 S78 S79 S80 S81 S82 S83 S84 S85 S86 S87 S88 S89 S90 S91 S92 S93 S94 S95 | L2 L4 S48 | L0 L28 S48 | L4 L6 S48 | L6 L8 S48 | L8 L10 S48 | L10 L12 S48 | L12 L14 S48 | L14 L48 S48 | L16 L18 S48 | L18 L20 S48 | L20 L22 S48 | L22 L24 S48 | L24 L26 S48 | L26 L28 S48 | L16 L48 S48